FakeTag_Fahrrad_v3 (Autodesk Fusion 360 design; units mm, degrees)
Autodesk Fusion 360 part; units mm, degrees
sketch "Sketch1" plane through (0, 0, 0) normal (0, 1, 0) x (1, 0, 0)
  line L0 (16.1, -19.1) -> (-16.1, -19.1)
  line L1 (-19.1, -16.1) -> (-19.1, 16.1)
  line L2 (-16.1, 19.1) -> (16.1, 19.1)
  line L3 (19.1, 16.1) -> (19.1, -16.1)
  line L4 (19.1, -19.1) -> (-19.1, 19.1) construction
  line L5 (-19.1, -19.1) -> (19.1, 19.1) construction
  arc A0 (-16.1, 19.1) -> (-19.1, 16.1) centre (-16.1, 16.1) ccw
  arc A1 (19.1, 16.1) -> (16.1, 19.1) centre (16.1, 16.1) ccw
  arc A2 (16.1, -19.1) -> (19.1, -16.1) centre (16.1, -16.1) ccw
  arc A3 (-19.1, -16.1) -> (-16.1, -19.1) centre (-16.1, -16.1) ccw
  line L6 (35.5, 5) -> (29.5, 5)
  arc A4 (29.5, 5) -> (29.5, -5) centre (29.5, 0) ccw
  line L7 (29.5, -5) -> (35.5, -5)
  arc A5 (35.5, -5) -> (35.5, 5) centre (35.5, 0) ccw
  line L8 (35.5, 0) -> (29.5, 0) construction
  line L9 (29.5, -3) -> (35.5, -3)
  arc A6 (35.5, -3) -> (35.5, 3) centre (35.5, 0) ccw
  line L10 (35.5, 3) -> (29.5, 3)
  arc A7 (29.5, 3) -> (29.5, -3) centre (29.5, 0) ccw
  line L11 (29.5, 0) -> (35.5, 0) construction
  arc A8 (-29.5, -5) -> (-29.5, 5) centre (-29.5, 0) ccw
  line L12 (-35.5, 0) -> (-29.5, 0) construction
  line L13 (-29.5, 3) -> (-35.5, 3)
  arc A9 (-29.5, -3) -> (-29.5, 3) centre (-29.5, 0) ccw
  line L14 (-35.5, -5) -> (-29.5, -5)
  line L15 (-29.5, 5) -> (-35.5, 5)
  arc A10 (-35.5, 3) -> (-35.5, -3) centre (-35.5, 0) ccw
  line L16 (-35.5, -3) -> (-29.5, -3)
  line L17 (-29.5, 0) -> (-35.5, 0) construction
  arc A11 (-35.5, 5) -> (-35.5, -5) centre (-35.5, 0) ccw
  ellipse E0 centre (0, 0) end of major axis (47.5, 0) minor radius 25.1
  line L18 (-47.5, 0) -> (47.5, 0) construction
  line L19 (0, -25.1) -> (0, 25.1) construction
  arc A12 (18.9, 16.1) -> (16.1, 18.9) centre (16.1, 16.1) ccw
  line L20 (-16.1, 18.9) -> (16.1, 18.9)
  arc A13 (-16.1, 18.9) -> (-18.9, 16.1) centre (-16.1, 16.1) ccw
  line L21 (-18.9, -16.1) -> (-18.9, 16.1)
  arc A14 (-18.9, -16.1) -> (-16.1, -18.9) centre (-16.1, -16.1) ccw
  line L22 (16.1, -18.9) -> (-16.1, -18.9)
  arc A15 (16.1, -18.9) -> (18.9, -16.1) centre (16.1, -16.1) ccw
  line L23 (18.9, 16.1) -> (18.9, -16.1)
  point P0 (32.5, 0)
  point P1 (32.5, 0)
  point P2 (-32.5, 0)
  point P3 (-32.5, 0)
  dimension "d1" = 38.2
  dimension "d2" = 3
  dimension "d5" = 38.2
  dimension "d6" = 3
  dimension "d7" = 3
  dimension "d12" = 32.5
  dimension "d15" = 10
  dimension "d16" = 6
  dimension "d17" = 10
  dimension "d18" = 6
  dimension "d19" = 32.5
  dimension "d22" = 3
  dimension "d23" = 3
  dimension "d24" = 6
  dimension "d25" = 12
  dimension "d26" = 0.2
  constraint horizontal L0
  constraint perpendicular L0 L1
  constraint parallel L0 L2
  constraint parallel L1 L3
  constraint coincident L4 E0.centre
  constraint coincident L5 E0.centre
  constraint coincident E0.centre origin
  constraint coincident L4.end L1
  constraint coincident L4.end L2
  constraint tangent L1 A0
  constraint tangent L2 A0
  constraint coincident L5.end L2
  constraint coincident L5.end L3
  constraint tangent L2 A1
  constraint tangent L3 A1
  constraint coincident L4.start L3
  constraint coincident L4.start L0
  constraint tangent L3 A2
  constraint tangent L0 A2
  constraint coincident L5.start L1
  constraint coincident L5.start L0
  constraint tangent L1 A3
  constraint tangent L0 A3
  constraint equal A2 A3
  constraint tangent L6 A4
  constraint tangent A4 L7
  constraint parallel L6 L7
  constraint tangent L7 A5
  constraint tangent L6 A5
  constraint horizontal L8
  constraint midpoint L8 P1
  constraint tangent L9 A6
  constraint tangent A6 L10
  constraint parallel L9 L10
  constraint tangent L10 A7
  constraint tangent L9 A7
  constraint parallel L8 L11
  constraint coincident P1 P0
  constraint midpoint L11 P1
  constraint tangent L15 A11
  constraint tangent L14 A11
  constraint parallel L14 L15
  constraint tangent A8 L14
  constraint tangent A8 L15
  constraint horizontal L17
  constraint midpoint P3 L17
  constraint tangent A9 L16
  constraint tangent L13 A9
  constraint parallel L13 L16
  constraint tangent L13 A10
  constraint tangent A10 L16
  constraint parallel L12 L17
  constraint coincident P3 P2
  constraint midpoint P3 L12
  constraint coincident E0 L18.start
  constraint coincident E0 L18.end
  constraint coincident E0 L19.start
  constraint coincident E0 L19.end
  constraint perpendicular L3 L18
  constraint coincident P1 L18
  constraint concentric A8 A9
  constraint concentric A4 A7
  measures "d1" distance of L5.start L4.end
  measures "d2" radius of A0
  measures "d5" distance of L1 L3
  measures "d6" radius of A1
  measures "d7" radius of A2
  measures "d12" distance of E0.centre P1
  measures "d15" diameter of A4
  measures "d16" diameter of A6
  measures "d17" diameter of A11
  measures "d18" diameter of A9
  measures "d19" distance of E0.centre P3
  measures "d22" distance of A5.centre P1
  measures "d23" distance of A8.centre P3
  measures "d24" distance of L2 L19.end
  measures "d25" distance of A5.centre L18.end
extrude "Extrude1" add sketch "Sketch1" against normal blind 3 contours L0 L1 L2 L3 A0 A1 A2 A3 | L6 A4 L7 A5 | A8 L14 L15 A11 | E0 | A12 L20 A13 L21 A14 L22 A15 L23 makes body 1
extrude "Extrude2" add sketch "Sketch1" along normal blind 2 contours A12 L20 A13 L21 A14 L22 A15 L23 bodies 1
ref_plane "WorkPlane1" through (0, 3, 0) normal (0, 1, 0) x (1, 0, 0)
sketch "Sketch3" plane through (0, 3, 0) normal (0, 1, 0) x (1, 0, 0)
  arc A0 (-29.5, -5) -> (-29.5, 5) centre (-29.5, 0) ccw
  line L0 (-35.5, -5) -> (-29.5, -5)
  arc A1 (-35.5, 5) -> (-35.5, -5) centre (-35.5, 0) ccw
  line L1 (-29.5, 5) -> (-35.5, 5)
  arc A2 (29.5, 5) -> (29.5, -5) centre (29.5, 0) ccw
  line L2 (29.5, -5) -> (35.5, -5)
  arc A3 (-35.5, 3) -> (-35.5, -3) centre (-35.5, 0) ccw
  line L3 (-35.5, -3) -> (-29.5, -3)
  arc A4 (-29.5, -3) -> (-29.5, 3) centre (-29.5, 0) ccw
  line L4 (-29.5, 3) -> (-35.5, 3)
  arc A5 (29.5, 3) -> (29.5, -3) centre (29.5, 0) ccw
  line L5 (35.5, 3) -> (29.5, 3)
  line L6 (29.5, -3) -> (35.5, -3)
  arc A6 (35.5, -3) -> (35.5, 3) centre (35.5, 0) ccw
  arc A7 (35.5, -5) -> (35.5, 5) centre (35.5, 0) ccw
  line L7 (35.5, 5) -> (29.5, 5)
  arc A8 (35.5, -4.85) -> (35.5, 4.85) centre (35.5, 0) ccw
  line L8 (35.5, 4.85) -> (29.5, 4.85)
  arc A9 (29.5, 4.85) -> (29.5, -4.85) centre (29.5, 0) ccw
  line L9 (29.5, -4.85) -> (35.5, -4.85)
  dimension "d49" = -0.15
extrude "Extrude3" add sketch "Sketch1" along normal blind 11.8 separate body contours L6 A4 L7 A5 | A8 L14 L15 A11 | E0 makes body 2
extrude "Extrude4" cut sketch "Sketch3" along normal blind 14 contours A0 L0 A1 L1 | A2 L2 A7 L7 | A8 L8 A9 L9 bodies 2
sketch "Sketch4" plane through (0, 11.8, 0) normal (0, 1, 0) x (-1, 0, 0)
  arc A0 (29.5, 5) -> (29.5, -5) centre (29.5, 0) ccw
  line L0 (29.5, 5) -> (35.5, 5)
  arc A1 (35.5, -5) -> (35.5, 5) centre (35.5, 0) ccw
  line L1 (35.5, -5) -> (29.5, -5)
  arc A2 (-35.5, 5) -> (-35.5, -5) centre (-35.5, 0) ccw
  line L2 (-35.5, 5) -> (-29.5, 5)
  arc A3 (-29.5, -5) -> (-29.5, 5) centre (-29.5, 0) ccw
  line L3 (-29.5, -5) -> (-35.5, -5)
  arc A4 (16.1, -19.1) -> (19.1, -16.1) centre (16.1, -16.1) ccw
  line L4 (16.1, -19.1) -> (-16.1, -19.1)
  arc A5 (-19.1, -16.1) -> (-16.1, -19.1) centre (-16.1, -16.1) ccw
  line L5 (-19.1, -16.1) -> (-19.1, 16.1)
  arc A6 (-16.1, 19.1) -> (-19.1, 16.1) centre (-16.1, 16.1) ccw
  line L6 (-16.1, 19.1) -> (16.1, 19.1)
  arc A7 (19.1, 16.1) -> (16.1, 19.1) centre (16.1, 16.1) ccw
  line L7 (19.1, 16.1) -> (19.1, -16.1)
  ellipse E0 centre (0, 0) end of major axis (-47.5, 0) minor radius 25.1
extrude "Extrude5" add sketch "Sketch4" along normal blind 2.5 contours A4 L4 A5 L5 A6 L6 A7 L7 | E0 bodies 2
fillet "Fillet1" radius 0.5 16 edges at (0, 0, 19.1) (-18.2213, 0, 18.2213) (-19.1, 0, 0) (-18.2213, 0, -18.2213) (0, 0, -19.1) (18.2213, 0, -18.2213) (19.1, 0, 0) (18.2213, 0, 18.2213) (-32.5, 0, 3) (-38.5, 0, 0) (-32.5, 0, -3) (-26.5, 0, 0) (32.5, 0, 3) (26.5, 0, 0) (32.5, 0, -3) (38.5, 0, 0) on bodies 2
fillet "Fillet2" radius 0.2 8 edges at (32.5, 14.3, -5) (40.5, 14.3, 0) (32.5, 14.3, 5) (24.5, 14.3, 0) (-32.5, 14.3, -5) (-24.5, 14.3, 0) (-32.5, 14.3, 5) (-40.5, 14.3, 0) on bodies 2
fillet "Fillet3" radius 1 1 edges at (-47.5, 14.3, 0) on bodies 2
fillet "Fillet4" radius 0.5 24 edges at (32.5, 0, 3) (26.5, 0, 0) (32.5, 0, -3) (38.5, 0, 0) (0, 2, -18.9) (-18.0799, 2, -18.0799) (-18.9, 2, 0) (-18.0799, 2, 18.0799) (0, 2, 18.9) (18.0799, 2, 18.0799) (18.9, 2, 0) (18.0799, 2, -18.0799) (-32.5, 0, 3) (-38.5, 0, 0) (-32.5, 0, -3) (-26.5, 0, 0) (-26.5, -3, 0) (-32.5, -3, -3) (-38.5, -3, 0) (-32.5, -3, 3) (38.5, -3, 0) (32.5, -3, -3) (26.5, -3, 0) (32.5, -3, 3) on bodies 1
fillet "Fillet5" radius 1 1 edges at (-47.5, -3, 0) on bodies 1
extrude "Extrude6" add sketch "Sketch3" along normal blind 6 separate body contours A5 L5 L6 A6 | A8 L8 A9 L9 makes body 3
fillet "Fillet6" radius 0.3 4 edges at (32.5, 3, 4.85) (40.35, 3, 0) (32.5, 3, -4.85) (24.65, 3, 0) on bodies 3
cylinder "CylinderPrimitive1" cut diameter 2.85 height -4 placed x (1, 0, 0) y (0, 0, -1) z (0, 1, 0) at (32.5, 9, 0) bodies 3
equation "d1 = tag_length"
equation "d2 = tag_radius"
equation "tag_length = 38.2 mm"
equation "tag_radius = 3 mm"
equation "d5 = tag_length"
equation "d6 = tag_radius"
equation "d7 = tag_radius"
equation "holder_holes = holder_screws + 1 mm"
equation "d12 = holder_abstand / 2"
equation "holder_abstand = 65 mm"
equation "holder_screws = 5 mm"
equation "d15 = holder_screws * 2"
equation "d16 = holder_holes"
equation "d17 = holder_screws * 2"
equation "d18 = holder_holes"
equation "d19 = holder_abstand / 2"
equation "d22 = holder_holes / 2"
equation "d23 = holder_holes / 2"
equation "d24 = holder_holes"
equation "d25 = holder_holes * 2"
equation "tag_height = 9.8 mm"
equation "d33 = tag_height + 2 mm"
